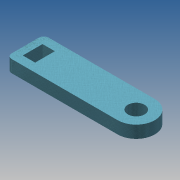
# Autodesk Inventor part: Kugellager-Schieber-Seite_M8Gewinde
Saved by Autodesk Inventor 2015 SP1 (Build 190203100, 203)
## iProperties
Created: 2015-01-28
Part Number: Kugellager-Schieber-Seite_M8Gewinde
Material: ABS-Kunststoff
Document SubType Name: Modeling
Designer: Marc
Density: 1.06 g/cm^3
Appearance: Gehont - dunkelgrau(1)
Mass: 3.36639 g
Surface Area: 19.9083 cm^2
Volume: 3.17584 cm^3
Author: Marc
Autodesk Inventor part; units mm, degrees
ref_plane "YZ Plane" through (0, 0, 0) normal (1, 0, 0) x (0, 1, 0)
ref_plane "XZ Plane" through (0, 0, 0) normal (0, 1, 0) x (-1, 0, 0)
ref_plane "XY Plane" through (0, 0, 0) normal (0, 0, 1) x (1, 0, 0)
sketch "Skizze1" plane through (0, 0, 0) normal (0, 0, 1) x (1, 0, 0)
  line L0 (0, -24.15) -> (0, 24.15) projected
  line L1 (-77.25, 0) -> (33, 0) projected
  circle A0 centre (-15.5, 15.5) radius 1.75
  circle A1 centre (15.5, 15.5) radius 1.75
  circle A2 centre (-15.5, -15.5) radius 1.75
  circle A3 centre (15.5, -15.5) radius 1.75
  circle A4 centre (-16.5, 0) radius 11
  circle A5 centre (0, 0) radius 5.5
  circle A6 centre (-16.5, 0) radius 3.4
  arc A7 (-16.5, -7.5) -> (-16.5, 7.5) centre (-16.5, 0) ccw
  line L2 (-16.5, 7.5) -> (-36.5, 7.5)
  line L3 (-36.5, 7.5) -> (-61.5, 7.5)
  line L4 (-61.5, 7.5) -> (-61.5, -7.5)
  line L5 (-61.5, -7.5) -> (-16.5, -7.5)
  dimension "d0" = 3.5
  dimension "d1" = 15.5
  dimension "d2" = 15.5
  dimension "d3" = 22
  dimension "d4" = 16.5
  dimension "d5" = 11
  dimension "d6" = 6.8
  dimension "d7" = 15
  dimension "d10" = 15
  dimension "d11" = 45
  constraints: 8 centre point, 8 end point, 3 coincident, 3 symmetric about line, 2 point on circle, 2 point on line, 2 tangent, 1 horizontal, 1 perpendicular, 3 other
  measures "d0" diameter of A0
  measures "d1" distance from line of L1 A0.centre
  measures "d2" distance from line of L0 A0.centre
  measures "d3" diameter of A4
  measures "d4" distance from line of L0 A4.centre
  measures "d5" diameter of A5
  measures "d6" diameter of A6
  measures "d7" diameter of A7
  measures "d10" distance of L3.end L4.end
  measures "d11" distance from line of L2.start L4
extrude "Extrusion1" add sketch "Skizze1" along normal blind 5 contours A7 L5 A4 L1 A6 | L1 A6 A4 L2 A7 | A4 L1 L4 L3 L2 | L5 L4 L1 A4
sketch "Skizze3" plane through (0, 0, 0) normal (0, 0, -1) x (-1, 0, 0)
  circle A0 centre (16.5, 0) radius 3.4 projected
  arc A1 (16.5, 7.5) -> (16.5, -7.5) centre (16.5, 0) ccw projected
  line L0 (16.5, -7.5) -> (61.5, -7.5) projected
  line L1 (61.5, -7.5) -> (61.5, 7.5) projected
  line L2 (61.5, 7.5) -> (16.5, 7.5) projected
  line L3 (58.5, -4) -> (53.5, -4)
  line L4 (53.5, -4) -> (53.5, 4)
  line L5 (53.5, 4) -> (58.5, 4)
  line L6 (58.5, 4) -> (58.5, -4)
  line L7 (73.8, 0) -> (-12.3, 0) projected
  point P0 (0, 0)
  dimension "d17" = 5
  dimension "d18" = 8
  dimension "d19" = 3
  constraints: 8 end point, 2 parallel, 1 horizontal, 1 perpendicular, 1 other
  measures "d17" distance of L4.end L5.end
  measures "d18" distance of L3.end L4.end
  measures "d19" distance between parallel lines of L1 L6
extrude "Extrusion3" cut sketch "Skizze3" against normal blind 5 contours L7 L6 L3 L4 | L4 L5 L6 L7
fillet "Rundung1" radius 2 2 edges at (-61.5, 7.5, 2.5) (-61.5, -7.5, 2.5)
